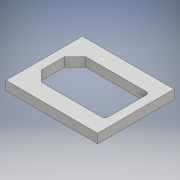
# Autodesk Inventor part: Estrutura - Tomada
Saved by Autodesk Inventor 2017 (Build 210142000, 142)
## iProperties
Created: 2020-09-27
Part Number: Estrutura - Tomada
Material: Generic
Document SubType Name: Modeling
Designer: ale
Density: 1 g/cm^3
Appearance: Default
Author: ale
Autodesk Inventor part; units mm, degrees
ref_plane "YZ Plane" through (0, 0, 0) normal (1, 0, 0) x (0, 1, 0)
ref_plane "XZ Plane" through (0, 0, 0) normal (0, 1, 0) x (-1, 0, 0)
ref_plane "XY Plane" through (0, 0, 0) normal (0, 0, 1) x (1, 0, 0)
sketch "Sketch1" plane through (0, 0, 0) normal (0, 0, 1) x (1, 0, 0)
  line L0 (-17.25, 14.5) -> (22.25, 14.5)
  line L1 (24.25, 12.5) -> (24.25, -12.5)
  line L2 (22.25, -14.5) -> (-17.25, -14.5)
  line L3 (-24.25, -7.5) -> (-24.25, 7.5)
  line L4 (-24.25, 14.5) -> (24.25, -14.5) construction
  line L5 (24.25, 14.5) -> (-24.25, -14.5) construction
  line L6 (-24.25, 7.5) -> (-17.25, 14.5)
  line L7 (-24.25, -7.5) -> (-17.25, -14.5)
  arc A0 (24.25, 12.5) -> (22.25, 14.5) centre (22.25, 12.5) ccw
  arc A1 (22.25, -14.5) -> (24.25, -12.5) centre (22.25, -12.5) ccw
  line L8 (-30, 25) -> (30, 25)
  line L9 (30, 25) -> (30, -25)
  line L10 (30, -25) -> (-30, -25)
  line L11 (-30, -25) -> (-30, 25)
  line L12 (-30, 25) -> (30, -25) construction
  line L13 (30, 25) -> (-30, -25) construction
  point P0 (0, 0)
  dimension "d0" = 48.5
  dimension "d1" = 29
  dimension "d3" = 7
  dimension "d4" = 7
  dimension "d5" = 7
  dimension "d6" = 7
  dimension "d7" = 2
  dimension "d8" = 60
  dimension "d9" = 50
  constraints: 28 end point, 8 point on line, 4 midpoint, 4 parallel, 4 point on circle, 4 tangent, 2 centre point, 2 horizontal, 2 perpendicular, 1 equal radius
  measures "d0" distance of L4.end L5.end
  measures "d1" distance of L5.start L4.end
  measures "d3" distance of L3.end L4.start
  measures "d4" distance of L0.start L4.start
  measures "d5" distance of L3.start L5.end
  measures "d6" distance of L2.end L5.end
  measures "d7" radius of A0
  measures "d8" distance of L9.end L10.end
  measures "d9" distance of L8.end L9.end
extrude "Extrusion1" add sketch "Sketch1" against normal blind 6
equation "\"d4\" = d3"
equation "\"d5\" = d3"
equation "\"d6\" = d5"
body "Solid1"
